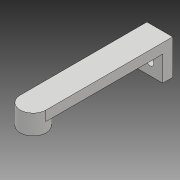
# Autodesk Inventor part: terminal_mount_front
Saved by Autodesk Inventor 2018 (Build 220112000, 112)
## iProperties
Created: 2017-06-03
Part Number: terminal_mount_front
Material: Generic
Document SubType Name: Modeling
Designer: AYUSH SHUKLA
Density: 1 g/cm^3
Appearance: Default
Author: AYUSH SHUKLA
Autodesk Inventor part; units mm, degrees
ref_plane "YZ Plane" through (0, 0, 0) normal (1, 0, 0) x (0, 1, 0)
ref_plane "XZ Plane" through (0, 0, 0) normal (0, 1, 0) x (-1, 0, 0)
ref_plane "XY Plane" through (0, 0, 0) normal (0, 0, 1) x (1, 0, 0)
sketch "Sketch1" plane through (0, 0, 0) normal (0, 1, 0) x (-1, 0, 0)
  line L0 (-6.5, -2.5) -> (6.5, -2.5)
  line L1 (6.5, -2.5) -> (6.5, 2.5)
  line L2 (6.5, 2.5) -> (-6.5, 2.5)
  line L3 (-6.5, 2.5) -> (-6.5, -2.5)
  line L4 (-6.5, -2.5) -> (6.5, 2.5) construction
  line L5 (6.5, -2.5) -> (-6.5, 2.5) construction
  point P0 (0, 0)
  dimension "d0" = 13
  dimension "d1" = 5
  constraints: 12 end point, 2 midpoint, 2 parallel, 1 horizontal, 1 perpendicular
  measures "d0" distance of L2.end L1.end
  measures "d1" distance of L1.end L0.end
extrude "Extrusion1" add sketch "Sketch1" along normal blind 70.4
sketch "Sketch2" plane through (0, 70.4, 0) normal (0, 1, 0) x (1, 0, 0)
  line L0 (6.5, 2.5) -> (6.5, -2.5) projected
  line L1 (6.5, -2.5) -> (-6.5, -2.5) projected
  line L2 (-6.5, -2.5) -> (-6.5, 2.5) projected
  line L3 (-6.5, 2.5) -> (6.5, 2.5) projected
  line L4 (-6.5, -2.5) -> (6.5, -2.5)
  line L5 (6.5, -2.5) -> (6.5, 15.2)
  line L6 (6.5, 15.2) -> (-6.5, 15.2)
  line L7 (-6.5, 15.2) -> (-6.5, -2.5)
  point P0 (0, 0)
  dimension "d4" = 17.7
  constraints: 8 end point, 2 parallel, 1 horizontal, 1 perpendicular
  measures "d4" distance of L5.end L4.end
extrude "Extrusion2" add sketch "Sketch2" against normal blind 5 contours L3 L7 L6 L5
fillet "Fillet1" radius 6.5 2 edges at (6.5, 0, 0) (-6.5, 0, 0)
sketch "Sketch3" plane through (6.5, 65.4, -2.5) normal (0, 0, -1) x (-1, 0, 0)
  arc A0 (0, -58.9) -> (13, -58.9) centre (6.5, -58.9) ccw projected
  line L0 (0, -58.9) -> (0, 0) projected
  line L1 (0, 0) -> (0, 5) projected
  line L2 (0, 5) -> (13, 5) projected
  line L3 (13, 5) -> (13, 0) projected
  line L4 (13, 0) -> (13, -58.9) projected
  line L5 (13, 0) -> (0, 0) projected
  circle A1 centre (6.5, -58.9) radius 6.5
  point P0 (6.5, -65.4)
  constraints: 1 centre point, 1 coincident, 1 tangent
extrude "Extrusion3" add sketch "Sketch3" along normal blind 5 contours A1 A0
sketch "Sketch4" plane through (0, 70.4, 0) normal (0, 1, 0) x (1, 0, 0)
  line L0 (6.5, -2.5) -> (-6.5, -2.5) projected
  line L1 (-6.5, -2.5) -> (-6.5, 15.2) projected
  line L2 (-6.5, 15.2) -> (6.5, 15.2) projected
  line L3 (6.5, 15.2) -> (6.5, -2.5) projected
  line L4 (6.5, -2.5) -> (-6.5, -2.5) projected
  line L5 (-6.5, -2.5) -> (-6.5, 15.2) projected
  line L6 (-6.5, 15.2) -> (6.5, 15.2) projected
  line L7 (6.5, 15.2) -> (6.5, -2.5) projected
  line L8 (-6.5, 2.5) -> (6.5, 2.5) projected
  circle A0 centre (0, 8.85) radius 2
  point P0 (0, 0)
  dimension "d10" = 4
  dimension "d11" = 6.35
  dimension "d12" = 6.5
  constraints: 1 centre point
  measures "d10" diameter of A0
  measures "d11" distance from line of L2 A0.centre
  measures "d12" distance from line of L1 A0.centre
extrude "Extrusion4" cut sketch "Sketch4" against normal up to surface (5 mm away) contours A0
body "Solid1"
